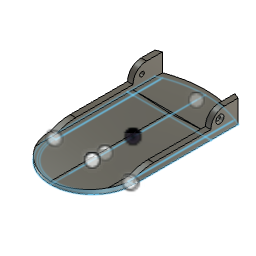
Wheelhouse rain deflector v7 (Autodesk Fusion 360 design; units mm, degrees)
Autodesk Fusion 360 part; units mm, degrees
note: some values were not read from the file. Chosen so that the rebuilt part matches the saved one: which sketch regions a step uses.
sketch "Sketch3" plane through (0, 0, 0) normal (0, 0, 1) x (1, 0, 0)
  line L0 (40, -45) -> (40, 72.5278)
  line L1 (-40, 70) -> (-40, -45)
  line L2 (0, 80) -> (0, -91)
  line L3 (-40, -45) -> (-40, 72.5278)
  line L4 (0, 70) -> (0, -70)
  line L5 (40, -45) -> (40, 70)
  line L6 (-46, 70) -> (-46, 40)
  line L7 (-46, 40) -> (-40, 40)
  line L8 (-40, 40) -> (-40, 70)
  line L9 (46, 70) -> (46, 40)
  line L10 (46, 40) -> (40, 40)
  line L11 (40, 40) -> (40, 70)
  arc A0 (46, 70) -> (-46, 70) centre (0, -30.8) ccw
  line L12 (-40, 40) -> (40, 40)
  line L13 (-46, 40) -> (-40, 40)
  line L14 (-40, 40) -> (-40, -45)
  line L15 (-40, -45) -> (-46, -45)
  line L16 (-46, -45) -> (-46, 40)
  line L17 (46, 40) -> (40, 40)
  line L18 (40, 40) -> (40, -45)
  line L19 (40, -45) -> (46, -45)
  line L20 (46, -45) -> (46, 40)
  arc A1 (-46, -45) -> (46, -45) centre (0, -45) ccw
  arc A2 (-43, -45) -> (43, -45) centre (0, -45) ccw
  arc A3 (-41, -45) -> (41, -45) centre (0, -45) ccw
  dimension "d29" = 80
  dimension "d31" = 6
  dimension "d32" = 30
  dimension "d33" = 6
  dimension "d34" = 30
  constraint parallel L0 L1
  constraint vertical L2
  constraint vertical L3
  constraint vertical L4
  constraint vertical L5
  constraint vertical L6
  constraint horizontal L7
  constraint vertical L8
  constraint vertical L9
  constraint horizontal L10
  constraint vertical L11
  constraint coincident L4.end L2
  constraint coincident A0 L2.start
  constraint coincident A0 L3.end
  constraint coincident L1.start L3
  constraint coincident A0 L0.end
  constraint coincident L5.end L0
  constraint perpendicular L5 L12
  constraint horizontal L13
  constraint vertical L14
  constraint horizontal L15
  constraint vertical L16
  constraint horizontal L17
  constraint vertical L18
  constraint horizontal L19
  constraint vertical L20
  constraint coincident A1 L2.end
  measures "d29" distance of L5.end L1.start
  measures "d31" distance of L1.start L6.start
  measures "d32" distance of L1.start L7.end
  measures "d33" distance of L5.end L9.start
  measures "d34" distance of L5.end L10.end
extrude "Extrude6" add sketch "Sketch3" along normal blind 5 contours L0 L2 L4 L5 L11 A0 L12 makes body 1
extrude "Extrude7" add sketch "Sketch3" along normal blind 5 separate body contours L1 L2 L3 L4 L8 A0 L12 makes body 2
chamfer "Chamfer1" distance 35 distance2 1.5 1 edges at (0, 60, 5) measured on face at (22.336, 52.2193, 5) on bodies 1
chamfer "Chamfer2" distance 35 distance2 1.5 1 edges at (0, 60, 5) measured on face at (-22.336, 52.2193, 5) on bodies 2
extrude "Extrude8" add sketch "Sketch3" along normal blind 25 contours L0 L5 L9 L10 L11 A0 L17 bodies 1
extrude "Extrude9" add sketch "Sketch3" along normal blind 25 contours L1 L3 L6 L7 L8 A0 L13 bodies 2
fillet "Fillet3" radius 15 1 edges at (-43, 40, 25) on bodies 2
fillet "Fillet4" radius 15 1 edges at (43, 40, 25) on bodies 1
extrude "Extrude10" add sketch "Sketch3" along normal blind 5 separate body contours L0 L2 L4 L5 L11 A0 L12 | L1 L2 L3 L4 L8 A0 L12 makes body 3
sketch "Sketch5" plane through (0, 0, 0) normal (1, 0, 0) x (0, 1, 0)
  circle A0 centre (0, 0) radius 2.5
  dimension "d54" = 5
  constraint coincident A0.centre origin
  measures "d54" diameter of A0
extrude "Extrude11" add sketch "Sketch5" along normal mid plane 100 separate body makes body 4
move_body "Move1" bodies 4 to x (1, 0, 0) y (0, 1, 0) z (0, 0, 1) at (0, 50, 15)
combine "Combine1" operation cut target body 2 tool bodies 4 keep tools
combine "Combine2" operation cut target body 1 tool bodies 4
chamfer "Chamfer3" distance 2 distance2 2 1 edges at (46, 47.6692, 15.904) measured on face at (46, 64.1574, 13.2091) on bodies 1
chamfer "Chamfer4" distance 2 distance2 2 1 edges at (-46, 47.6692, 14.096) measured on face at (-46, 64.1574, 13.2091) on bodies 2
combine "Combine3" operation cut target body 1 tool bodies 2 keep tools
combine "Combine4" operation cut target body 2 tool bodies 1 keep tools
extrude "Extrude13" cut sketch "Sketch3" along normal blind 1 contours L1 L2 L3 L4 L12 L14 L15 A3 bodies 1 2
extrude "Extrude14" add sketch "Sketch3" along normal blind 5 contours L0 L2 L4 L5 L12 L18 L19 A3 | L2 L19 A2 A3 | L2 L19 A1 A2 bodies 1 2 3
chamfer "Chamfer5" distance 40 distance2 2 1 edges at (0, -25.5, 5) measured on face at (13.3333, -32, 5) on bodies 1
extrude "Extrude15" add sketch "Sketch3" along normal blind 5 separate body contours L1 L2 L3 L4 L12 L14 L15 A3 | L2 L15 A2 A3 | L2 L15 A1 A2 makes body 5
chamfer "Chamfer6" distance 40 distance2 2 1 edges at (0, -25.5, 5) measured on face at (-13.3333, -25, 5) on bodies 5
extrude "Extrude16" add sketch "Sketch3" along normal blind 10 contours L0 L5 L10 L17 L18 L19 L20 | L1 L3 L7 L13 L14 L15 L16 bodies 1 5
fillet "Fillet5" radius 50 2 edges at (43, -45, 10) (-43, -45, 10) on bodies 1
extrude "Extrude17" cut sketch "Sketch3" along normal blind 1 contours L2 L19 A2 A3 | L2 L15 A2 A3 bodies 1
